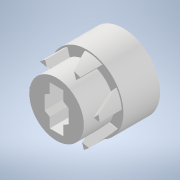
# Autodesk Inventor part: female mixing head
Saved by Autodesk Inventor 2022 (Build 260153000, 153)
## iProperties
Created: 2022-05-06
Part Number: female mixing head
Material: Generic
Document SubType Name: Modeling
Designer: efred
Density: 1 g/cm^3
Appearance: Default
Author: efred
Autodesk Inventor part; units mm, degrees
ref_plane "YZ Plane" through (0, 0, 0) normal (1, 0, 0) x (0, 1, 0)
ref_plane "XZ Plane" through (0, 0, 0) normal (0, 1, 0) x (-1, 0, 0)
ref_plane "XY Plane" through (0, 0, 0) normal (0, 0, 1) x (1, 0, 0)
sketch "Sketch1" plane through (0, 0, 0) normal (0, 0, 1) x (1, 0, 0)
  line L0 (4.5981, -1.5) -> (6.005, -1.5) construction
  arc A0 (-0.5981, -1.5) -> (4.5981, -1.5) centre (2, 0) ccw construction
  line L1 (-1.995, -1.5) -> (-0.5981, -1.5) construction
  line L2 (-1.995, 1.5) -> (-1.995, -1.5) construction
  line L3 (-0.5981, 1.5) -> (-1.995, 1.5) construction
  arc A1 (4.5981, 1.5) -> (-0.5981, 1.5) centre (2, 0) ccw construction
  line L4 (6.005, 1.5) -> (4.5981, 1.5) construction
  line L5 (6.005, -1.5) -> (6.005, 1.5) construction
  spline S0 degree 3 poles (-3.0757, 5.5216) (-3.0769, 5.5129) (-3.0781, 5.5043) (-3.136, 5.095) (-3.2274, 4.6999) (-3.4287, 4.0986) (-3.5391, 3.8305) (-3.8095, 3.3218) (-3.9701, 3.0814) (-4.4047, 2.5587) (-4.7883, 2.2395) (-5.1813, 2.0487) (-5.2004, 2.0397) (-5.2198, 2.0308) knots 0 0 0 0 0.005934 0.005934 0.28157 0.28157 0.478136 0.478136 0.674702 0.674702 0.984411 0.984411 1 1 1 1 construction
  arc A2 (-5.2198, 2.0308) -> (-3.0757, 5.5216) centre (2, 0) ccw construction
  arc A3 (5.4661, 6.0816) -> (1.3492, 6.9697) centre (2, 0) ccw construction
  line L6 (4.4276, 4.9352) -> (5.4661, 6.0816) construction
  arc A4 (6.672, 2.9021) -> (4.4276, 4.9352) centre (2, 0) ccw construction
  line L7 (7.7105, 4.0485) -> (6.672, 2.9021) construction
  arc A5 (8.9999, 0.0391) -> (7.7105, 4.0485) centre (2, 0) ccw construction
  line L8 (7.4879, 0.3652) -> (8.9999, 0.0391) construction
  arc A6 (6.8493, -2.5951) -> (7.4879, 0.3652) centre (2, 0) ccw construction
  line L9 (8.3613, -2.9212) -> (6.8493, -2.5951) construction
  arc A7 (5.5338, -6.0425) -> (8.3613, -2.9212) centre (2, 0) ccw construction
  line L10 (5.0602, -4.57) -> (5.5338, -6.0425) construction
  arc A8 (2.1773, -5.4971) -> (5.0602, -4.57) centre (2, 0) ccw construction
  line L11 (2.6508, -6.9697) -> (2.1773, -5.4971) construction
  arc A9 (-1.4661, -6.0816) -> (2.6508, -6.9697) centre (2, 0) ccw construction
  line L12 (-0.4276, -4.9352) -> (-1.4661, -6.0816) construction
  arc A10 (-2.672, -2.9021) -> (-0.4276, -4.9352) centre (2, 0) ccw construction
  line L13 (-3.7105, -4.0485) -> (-2.672, -2.9021) construction
  arc A11 (-4.9999, -0.0391) -> (-3.7105, -4.0485) centre (2, 0) ccw construction
  line L14 (-3.4879, -0.3652) -> (-4.9999, -0.0391) construction
  arc A12 (-2.8493, 2.5951) -> (-3.4879, -0.3652) centre (2, 0) ccw construction
  line L15 (-4.3613, 2.9212) -> (-2.8493, 2.5951) construction
  arc A13 (-1.5338, 6.0425) -> (-4.3613, 2.9212) centre (2, 0) ccw construction
  line L16 (-1.0602, 4.57) -> (-1.5338, 6.0425) construction
  arc A14 (1.8227, 5.4971) -> (-1.0602, 4.57) centre (2, 0) ccw construction
  line L17 (1.3492, 6.9697) -> (1.8227, 5.4971) construction
  circle A15 centre (2, 0) radius 7
  line L18 (-0.4799, 1.3) -> (-1.795, 1.3)
  line L19 (-1.795, 1.3) -> (-1.795, -1.3)
  line L20 (-1.795, -1.3) -> (-0.4799, -1.3)
  arc A16 (-0.4799, -1.3) -> (4.4799, -1.3) centre (2, 0) ccw
  line L21 (4.4799, -1.3) -> (5.805, -1.3)
  line L22 (5.805, -1.3) -> (5.805, 1.3)
  line L23 (5.805, 1.3) -> (4.4799, 1.3)
  arc A17 (4.4799, 1.3) -> (-0.4799, 1.3) centre (2, 0) ccw
  point P0 (0, 0)
  dimension "d1" = 0.5
  dimension "d15" = 0.2
  constraints: 12 end point, 4 point on circle, 3 centre point, 1 coincident, 7 other
  measures "d1" radial gap between concentric circles of A15 A2
  measures "d15" radial gap between concentric circles of A1 A17
ref_plane "Work Plane1" through (-23.125, -26, 7) normal (0, 0, 1) x (1, 0, 0)
extrude "Extrusion1" add sketch "Sketch1" along normal up to surface (7 mm away)
sketch "Sketch2" plane through (2, 0, 7) normal (0, 0, 1) x (1, 0, 0)
  arc A0 (3.4661, 6.0816) -> (-0.6508, 6.9697) centre (0, 0) ccw construction
  line L0 (2.4276, 4.9352) -> (3.4661, 6.0816) construction
  arc A1 (4.672, 2.9021) -> (2.4276, 4.9352) centre (0, 0) ccw construction
  line L1 (5.7105, 4.0485) -> (4.672, 2.9021) construction
  arc A2 (6.9999, 0.0391) -> (5.7105, 4.0485) centre (0, 0) ccw construction
  line L2 (5.4879, 0.3652) -> (6.9999, 0.0391) construction
  arc A3 (4.8493, -2.5951) -> (5.4879, 0.3652) centre (0, 0) ccw construction
  line L3 (6.3613, -2.9212) -> (4.8493, -2.5951) construction
  arc A4 (3.5338, -6.0425) -> (6.3613, -2.9212) centre (0, 0) ccw construction
  line L4 (3.0602, -4.57) -> (3.5338, -6.0425) construction
  arc A5 (0.1773, -5.4971) -> (3.0602, -4.57) centre (0, 0) ccw construction
  line L5 (0.6508, -6.9697) -> (0.1773, -5.4971) construction
  arc A6 (-3.4661, -6.0816) -> (0.6508, -6.9697) centre (0, 0) ccw construction
  line L6 (-2.4276, -4.9352) -> (-3.4661, -6.0816) construction
  arc A7 (-4.672, -2.9021) -> (-2.4276, -4.9352) centre (0, 0) ccw construction
  line L7 (-5.7105, -4.0485) -> (-4.672, -2.9021) construction
  arc A8 (-6.9999, -0.0391) -> (-5.7105, -4.0485) centre (0, 0) ccw construction
  line L8 (-5.4879, -0.3652) -> (-6.9999, -0.0391) construction
  arc A9 (-4.8493, 2.5951) -> (-5.4879, -0.3652) centre (0, 0) ccw construction
  line L9 (-6.3613, 2.9212) -> (-4.8493, 2.5951) construction
  arc A10 (-3.5338, 6.0425) -> (-6.3613, 2.9212) centre (0, 0) ccw construction
  line L10 (-3.0602, 4.57) -> (-3.5338, 6.0425) construction
  arc A11 (-0.1773, 5.4971) -> (-3.0602, 4.57) centre (0, 0) ccw construction
  line L11 (-0.6508, 6.9697) -> (-0.1773, 5.4971) construction
  circle A12 centre (0, 0) radius 7 construction
  line L12 (-3.219, 4.0839) -> (-3.7016, 5.5846)
  arc A13 (-3.7016, 5.5846) -> (-5.9222, 3.1334) centre (0, 0) ccw
  line L13 (-5.9222, 3.1334) -> (-4.3812, 2.801)
  arc A14 (-4.3812, 2.801) -> (-5.1462, -0.7458) centre (0, 0) ccw
  line L14 (-5.1462, -0.7458) -> (-6.6872, -0.4134)
  arc A15 (-6.6872, -0.4134) -> (-5.6747, -3.562) centre (0, 0) ccw
  line L15 (-5.6747, -3.562) -> (-4.6163, -2.3937)
  arc A16 (-4.6163, -2.3937) -> (-1.9272, -4.8297) centre (0, 0) ccw
  line L16 (-1.9272, -4.8297) -> (-2.9856, -5.998)
  arc A17 (-2.9856, -5.998) -> (0.2475, -6.6954) centre (0, 0) ccw
  line L17 (0.2475, -6.6954) -> (-0.2351, -5.1947)
  arc A18 (-0.2351, -5.1947) -> (3.219, -4.0839) centre (0, 0) ccw
  line L18 (3.219, -4.0839) -> (3.7016, -5.5846)
  arc A19 (3.7016, -5.5846) -> (5.9222, -3.1334) centre (0, 0) ccw
  line L19 (5.9222, -3.1334) -> (4.3812, -2.801)
  arc A20 (4.3812, -2.801) -> (5.1462, 0.7458) centre (0, 0) ccw
  line L20 (5.1462, 0.7458) -> (6.6872, 0.4134)
  arc A21 (6.6872, 0.4134) -> (5.6747, 3.562) centre (0, 0) ccw
  line L21 (5.6747, 3.562) -> (4.6163, 2.3937)
  arc A22 (4.6163, 2.3937) -> (1.9272, 4.8297) centre (0, 0) ccw
  line L22 (1.9272, 4.8297) -> (2.9856, 5.998)
  arc A23 (2.9856, 5.998) -> (-0.2475, 6.6954) centre (0, 0) ccw
  line L23 (-0.2475, 6.6954) -> (0.2351, 5.1947)
  arc A24 (0.2351, 5.1947) -> (-3.219, 4.0839) centre (0, 0) ccw
  line L24 (-2.4799, 1.3) -> (-3.795, 1.3) projected
  arc A25 (2.4799, 1.3) -> (-2.4799, 1.3) centre (0, 0) ccw projected
  line L25 (3.805, 1.3) -> (2.4799, 1.3) projected
  line L26 (2.4799, -1.3) -> (3.805, -1.3) projected
  arc A26 (-2.4799, -1.3) -> (2.4799, -1.3) centre (0, 0) ccw projected
  line L27 (-3.795, -1.3) -> (-2.4799, -1.3) projected
  line L28 (-3.795, 1.3) -> (-3.795, -1.3) projected
  circle A27 centre (0, 0) radius 7 construction
  line L29 (2.4799, -1.3) -> (3.805, -1.3) projected
  arc A28 (-2.4799, -1.3) -> (2.4799, -1.3) centre (0, 0) ccw projected
  line L30 (-3.795, -1.3) -> (-2.4799, -1.3) projected
  line L31 (-3.795, 1.3) -> (-3.795, -1.3) projected
  line L32 (-2.4799, 1.3) -> (-3.795, 1.3) projected
  arc A29 (2.4799, 1.3) -> (-2.4799, 1.3) centre (0, 0) ccw projected
  line L33 (3.805, 1.3) -> (2.4799, 1.3) projected
  line L34 (3.805, -1.3) -> (3.805, 1.3) projected
  line L35 (3.805, -1.3) -> (3.805, 1.3) projected
  point P0 (-2, 0)
  dimension "d4" = 0.3
  constraints: 24 end point, 24 point on circle, 12 centre point, 23 other
  measures "d4" radial gap between concentric circles of A11 A24
ref_plane "Work Plane2" through (-8.1566, -8.2837, 12.7484) normal (0, 0, -1) x (0.2108593, 0.9775164, 0)
extrude "Extrusion2" add sketch "Sketch2" along normal up to surface (5.7484 mm away) contours A24 L23 A23 L22 A22 L21 A21 L20 A20 L19 A19 L18 A18 L17 A17 L16 A16 L15 A15 L14 A14 L13 A13 L12 | A25 L25 L34 L26 A26 L27 L28 L24
chamfer "Chamfer1" distance 2.6 angle 65 6 edges at (2.0062, -5.9451, 12.7484) (7.1517, -2.9672, 12.7484) (7.1455, 2.9779, 12.7484) (1.9938, 5.9451, 12.7484) (-3.1517, 2.9672, 12.7484) (-3.1455, -2.9779, 12.7484) measured on face at (2.4698, 6.0981, 12.7484) measured on face at (1.5302, -6.0981, 12.7484) measured on face at (7.0462, -3.4559, 12.7484) measured on face at (-3.0462, 3.4559, 12.7484) measured on face at (7.516, 2.6422, 12.7484) measured on face at (-3.516, -2.6422, 12.7484)
sketch "Sketch3" plane through (-0.6591, -6.1497, 12.7484) normal (0, 0, 1) x (0.9519837, 0.3061487, 0)
  arc A0 (-0.2643, 0.2443) -> (2.6, -1.4094) centre (4.4142, 5.0403) ccw projected
  line L0 (2.6, -1.4094) -> (2.6, 0.1671) projected
  line L1 (-0.2643, 0.2443) -> (1.1009, 1.0326) projected
  circle A1 centre (4.4142, 5.0403) radius 5.2 projected
  point P0 (2.5102, 5.6526)
  point P1 (-0.7133, 4.1748)
  point P2 (6.2284, 0.1671)
  point P3 (1.6734, -1.0734)
  point P4 (1.1009, 1.0326)
extrude "Extrusion3" cut sketch "Sketch3" against normal blind 1.5 contours L1 A1 L0 A0
pattern_circular "Circular Pattern1" count 6 over 360 about axis through (2, 0, 0) along (0, 0, 1) of "Extrusion3"
sketch "Sketch4" plane through (2, 0, 12.7484) normal (0, 0, 1) x (1, 0, 0)
  line L0 (-2, -1.1547) -> (-1, -1.7321) construction
  line L1 (-1, -1.7321) -> (-1, -3.5) construction
  line L2 (-1, -3.5) -> (1, -3.5) construction
  line L3 (1, -3.5) -> (1, -1.7321) construction
  line L4 (1, -1.7321) -> (2, -1.1547) construction
  line L5 (2, -1.1547) -> (2, 1.1547) construction
  line L6 (2, 1.1547) -> (1, 1.7321) construction
  line L7 (1, 1.7321) -> (1, 3.5) construction
  line L8 (1, 3.5) -> (-1, 3.5) construction
  line L9 (-1, 3.5) -> (-1, 1.7321) construction
  line L10 (-1, 1.7321) -> (-2, 1.1547) construction
  line L11 (-2, 1.1547) -> (-2, -1.1547) construction
  line L12 (-1.3, -3.8) -> (-1.3, -1.9053)
  line L13 (-1.3, -1.9053) -> (-2.3, -1.3279)
  line L14 (-2.3, -1.3279) -> (-2.3, 1.3279)
  line L15 (-2.3, 1.3279) -> (-1.3, 1.9053)
  line L16 (-1.3, 1.9053) -> (-1.3, 3.8)
  line L17 (-1.3, 3.8) -> (1.3, 3.8)
  line L18 (1.3, 3.8) -> (1.3, 1.9053)
  line L19 (1.3, 1.9053) -> (2.3, 1.3279)
  line L20 (2.3, 1.3279) -> (2.3, -1.3279)
  line L21 (2.3, -1.3279) -> (1.3, -1.9053)
  line L22 (1.3, -1.9053) -> (1.3, -3.8)
  line L23 (1.3, -3.8) -> (-1.3, -3.8)
  circle A0 centre (0, 0) radius 5.2 construction
  line L24 (-4.6163, -2.3937) -> (-5.6747, -3.562) construction
  circle A1 centre (0, 0) radius 7 construction
  arc A2 (2.4799, 1.3) -> (-2.4799, 1.3) centre (0, 0) ccw projected
  line L25 (-3.795, 1.3) -> (-2.4799, 1.3) projected
  line L26 (-3.795, -1.3) -> (-3.795, 1.3) projected
  line L27 (-2.4799, -1.3) -> (-3.795, -1.3) projected
  arc A3 (-2.4799, -1.3) -> (2.4799, -1.3) centre (0, 0) ccw projected
  line L28 (3.805, -1.3) -> (2.4799, -1.3) projected
  line L29 (3.805, 1.3) -> (3.805, -1.3) projected
  line L30 (2.4799, 1.3) -> (3.805, 1.3) projected
  point P0 (1.3, -2.4799)
  point P1 (1.3, 2.4799)
  point P2 (-1.3, 2.4799)
  point P3 (-1.3, -2.4799)
  dimension "d19" = 0.3
  constraints: 24 end point, 12 other
  measures "d19" distance between parallel lines of L1 L12
ref_plane "Work Plane3" through (-2, -3.5, 6.9) normal (0, 0, 1) x (1, 0, 0)
extrude "Extrusion4" cut sketch "Sketch4" against normal up to surface (5.8484 mm away)
body "Solid1"
